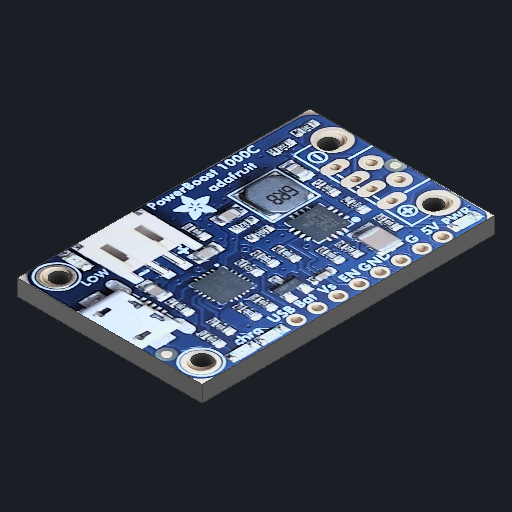
# Autodesk Inventor part: powerboost
Saved by Autodesk Inventor 2026.2 (Build 302298000, 298)
## iProperties
Created: 2025-06-04
Part Number: powerboost
Material: Generic
Document SubType Name: Modeling
Designer: cdavi
Density: 1 g/cm^3
Appearance: Default
Mass: 1.62993 g
Surface Area: 19.1644 cm^2
Volume: 1.62993 cm^3
Author: cdavi
Autodesk Inventor part; units mm, degrees
ref_plane "YZ Plane" through (0, 0, 0) normal (1, 0, 0) x (0, 1, 0)
ref_plane "XZ Plane" through (0, 0, 0) normal (0, 1, 0) x (-1, 0, 0)
ref_plane "XY Plane" through (0, 0, 0) normal (0, 0, 1) x (1, 0, 0)
sketch "Sketch1" plane through (0, 0, 0) normal (0, 1, 0) x (-1, 0, 0)
  line L0 (-11.43, 18.1) -> (11.43, 18.1)
  line L1 (11.43, 18.1) -> (11.43, -18.1)
  line L2 (11.43, -18.1) -> (-11.43, -18.1)
  line L3 (-11.43, -18.1) -> (-11.43, 18.1)
  line L4 (-11.43, 18.1) -> (11.43, -18.1) construction
  line L5 (11.43, 18.1) -> (-11.43, -18.1) construction
  line L6 (-8.825, 15.5) -> (8.825, 15.5) construction
  line L7 (8.825, 15.5) -> (8.825, -15.5) construction
  line L8 (8.825, -15.5) -> (-8.825, -15.5) construction
  line L9 (-8.825, -15.5) -> (-8.825, 15.5) construction
  line L10 (-8.825, 15.5) -> (8.825, -15.5) construction
  line L11 (8.825, 15.5) -> (-8.825, -15.5) construction
  circle A0 centre (8.825, 15.5) radius 1
  circle A1 centre (-8.825, 15.5) radius 1
  circle A2 centre (6.5, -15.5) radius 1
  line L12 (0, 0) -> (0, -18.1)
  circle A3 centre (-6.5, -15.5) radius 1
  dimension "d0" = 22.86
  dimension "d1" = 36.2
  dimension "d2" = 17.65
  dimension "d3" = 31
  dimension "d4" = 6.5
  dimension "d5" = 2
  dimension "d6" = 2
  dimension "d7" = 2
  constraints: 26 end point, 5 midpoint, 4 centre point, 4 parallel, 2 coincident, 2 horizontal, 2 perpendicular, 1 point on line, 1 symmetric about line, 1 other
  measures "d0" distance of L0.start L0.end
  measures "d1" distance of L0.end L1.end
  measures "d2" distance of L7.end L8.end
  measures "d3" distance of L6.end L7.end
  measures "d4" distance from line of L12 A2.centre
  measures "d5" diameter of A2
  measures "d6" diameter of A0
  measures "d7" diameter of A1
extrude "Extrusion1" add sketch "Sketch1" along normal blind 2
sketch "Sketch2" plane through (0, 2, 0) normal (0, 1, 0) x (1, 0, 0)
  line L0 (-11.43, 18.1) -> (11.3685, 18.1) construction
  line L1 (11.3685, 18.1) -> (11.3685, -18.1704) construction
  line L2 (11.3685, -18.1704) -> (-11.43, -18.1704) construction
  line L3 (-11.43, -18.1704) -> (-11.43, 18.1) construction
  point P0 (0, 0)
  constraints: 1 coincident, 1 vertical, 2 other
decal "Decal1"
body "Solid1"
